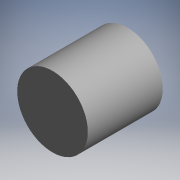
# Autodesk Inventor part: gearbox
Saved by Autodesk Inventor 2019.4 (Build 234330000, 330)
## iProperties
Created: 2020-06-20
Part Number: gearbox
Material: Generic
Document SubType Name: Modeling
Designer: Jorge
Density: 1 g/cm^3
Appearance: Default
Author: Jorge
Autodesk Inventor part; units mm, degrees
ref_plane "YZ Plane" through (0, 0, 0) normal (1, 0, 0) x (0, 1, 0)
ref_plane "XZ Plane" through (0, 0, 0) normal (0, 1, 0) x (-1, 0, 0)
ref_plane "XY Plane" through (0, 0, 0) normal (0, 0, 1) x (1, 0, 0)
sketch "Sketch1" plane through (0, 0, 0) normal (0, 0, 1) x (1, 0, 0)
  circle A0 centre (0, 0) radius 12.25
  dimension "d0" = 24.5
  constraints: 1 centre point, 1 coincident
  measures "d0" diameter of A0
extrude "Extrusion1" add sketch "Sketch1" along normal blind 26
chamfer "Chamfer1" distance 0.5 angle 45 1 edges at (-12.25, 0, 0)
chamfer "Chamfer2" distance 0.5 angle 45 1 edges at (-12.25, 0, 26)
body "Solid1"
